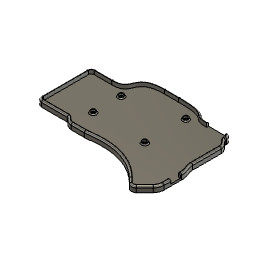
case (Autodesk Fusion 360 design; units mm, degrees)
Autodesk Fusion 360 part; units mm, degrees
note: some values were not read from the file. Chosen so that the rebuilt part matches the saved one: which bodies a step acts on; which pieces of a blend or face edit are solid. Set by a fixed rule: which sketch regions a step uses; the direction of a hole.
sketch "holes" plane through (0, 0, 0) normal (0, 1, 0) x (1, 0, 0)
  line L0 (126.0404, -106.5892) -> (126.0404, -96.5892)
  line L1 (157.8502, -159.4086) -> (150.6767, -159.4086)
  line L2 (126.0404, -96.5892) -> (146.0404, -96.5892)
  line L3 (150.6767, -159.4086) -> (150.6767, -169.4086)
  line L4 (146.0404, -106.5892) -> (126.0404, -106.5892)
  line L5 (150.6767, -169.4086) -> (157.8502, -169.4086)
  line L6 (146.0404, -96.5892) -> (146.0404, -106.5892)
  circle A0 centre (145.3008, -163.4257) radius 0.6
  circle A1 centre (145.3008, -165.1757) radius 0.6
  circle A2 centre (54.3208, -145.8157) radius 2.5
  circle A3 centre (108.3208, -146.3157) radius 2.5
  circle A4 centre (54.3208, -116.8157) radius 2.5
  line L7 (38.8208, -162.5657) -> (47.1808, -162.5657)
  spline S0 degree 3 poles (47.1808, -162.5657) (51.7408, -162.5657) (51.7408, -167.5657) (56.3208, -167.5657) knots 1 1 1 1 2 2 2 2
  line L8 (56.3208, -167.5657) -> (69.8508, -167.5657)
  spline S1 degree 3 poles (69.8508, -167.5657) (75.9008, -167.5657) (75.8208, -166.3157) (88.3208, -166.3157) (106.4584, -166.3157) (123.8522, -173.5257) (136.6708, -186.3576) knots 3 3 3 3 4 4 4 5 5 5 5
  line L9 (136.6708, -186.3576) -> (141.4208, -191.1076)
  spline S2 degree 3 poles (141.4208, -191.1076) (142.2162, -191.8832) (143.4896, -191.8677) (144.266, -191.073) knots 6 6 6 6 7 7 7 7
  line L10 (144.266, -191.073) -> (153.0169, -182.3192)
  spline S3 degree 3 poles (153.0169, -182.3192) (154.5362, -180.8058) (155.392, -178.7508) (155.3961, -176.6064) knots 8 8 8 8 9 9 9 9
  line L11 (155.3961, -176.6064) -> (155.3961, -158.2827)
  spline S4 degree 3 poles (155.3961, -158.2827) (155.3961, -150.8157) (152.3208, -150.8157) (152.3208, -143.8257) knots 10 10 10 10 11 11 11 11
  line L12 (152.3208, -143.8257) -> (152.3208, -114.1112)
  spline S5 degree 3 poles (152.3208, -114.1112) (152.3208, -110.3657) (146.8208, -108.1957) (146.8208, -104.4757) knots 12 12 12 12 13 13 13 13
  line L13 (146.8208, -104.4757) -> (146.8208, -103.0657)
  spline S6 degree 3 poles (146.8208, -103.0657) (146.8208, -101.9611) (145.9254, -101.0657) (144.8208, -101.0657) knots 14 14 14 14 15 15 15 15
  line L14 (144.8208, -101.0657) -> (126.8208, -101.0657)
  spline S7 degree 3 poles (126.8208, -101.0657) (106.3208, -101.0657) (123.3208, -93.0657) (89.0708, -93.0657) knots 17 17 17 17 18 18 18 18
  line L15 (89.0708, -93.0657) -> (74.3308, -93.0657)
  spline S8 degree 3 poles (74.3308, -93.0657) (43.8208, -93.0657) (61.8208, -111.8157) (38.8208, -112.0657) knots 19 19 19 19 20 20 20 20
  spline S9 degree 3 poles (38.8208, -112.0657) (37.7162, -112.0657) (36.8208, -112.9611) (36.8208, -114.0657) knots 20 20 20 20 21 21 21 21
  line L16 (36.8208, -114.0657) -> (36.8208, -114.5657)
  spline S10 degree 3 poles (36.8208, -114.5657) (36.8208, -114.8418) (36.5969, -115.0657) (36.0446, -115.0657) (35.8208, -114.8418) (35.8208, -114.5657) knots 23 23 23 23 24 24 25 25 25 25
  line L17 (35.8208, -114.5657) -> (35.8208, -114.0657)
  spline S11 degree 3 poles (35.8208, -114.0657) (35.8208, -112.9611) (34.9253, -112.0657) (33.8208, -112.0657) knots 26 26 26 26 27 27 27 27
  line L18 (33.8208, -112.0657) -> (20.5708, -112.0657)
  spline S12 degree 3 poles (20.5708, -112.0657) (19.4662, -112.0657) (18.5708, -112.9611) (18.5708, -114.0657) knots 29 29 29 29 30 30 30 30
  line L19 (18.5708, -114.0657) -> (18.5708, -160.5657)
  spline S13 degree 3 poles (18.5708, -160.5657) (18.5708, -161.6703) (19.4662, -162.5657) (20.5708, -162.5657) knots 32 32 32 32 33 33 33 33
  line L20 (20.5708, -162.5657) -> (33.8208, -162.5657)
  spline S14 degree 3 poles (33.8208, -162.5657) (34.9253, -162.5657) (35.8208, -161.6703) (35.8208, -160.5657) knots 35 35 35 35 36 36 36 36
  line L21 (35.8208, -160.5657) -> (35.8208, -160.0657)
  spline S15 degree 3 poles (35.8208, -160.0657) (35.8208, -159.7895) (36.0446, -159.5657) (36.5969, -159.5657) (36.8208, -159.7895) (36.8208, -160.0657) knots 38 38 38 38 39 39 40 40 40 40
  line L22 (36.8208, -160.0657) -> (36.8208, -160.5657)
  spline S16 degree 3 poles (36.8208, -160.5657) (36.8208, -161.6703) (37.7162, -162.5657) (38.8208, -162.5657) knots 41 41 41 41 42 42 42 42
  circle A5 centre (108.3208, -103.8157) radius 2.5
  line L23 (150.6767, -159.4086) -> (162.9306, -159.4086)
  line L24 (162.9306, -159.4086) -> (162.9306, -169.4086)
  line L25 (162.9306, -169.4086) -> (150.6767, -169.4086)
  line L26 (150.6767, -169.4086) -> (150.6767, -159.4086)
  dimension "d39" = 10
  constraint horizontal L23
  constraint vertical L24
  constraint horizontal L25
  constraint vertical L26
  measures "d39" distance of L1.end L3.end
extrude "Extrude7" add sketch "holes" along normal blind 4 contours A2 | A3 | A4 | A5 makes body 1 at (110.2359, 2.6667, 144.7087) makes body 2 at (56.8177, 2.6667, 116.9403) makes body 3 at (52.3279, 2.6667, 147.3252) makes body 4 at (106.328, 2.6667, 105.3252)
hole "Hole1" at (108.3208, 0, 103.8157) at (108.3208, 0, 146.3157) at (54.3208, 0, 116.8157) at (54.3208, 0, 145.8157) direction (0, 1, 0) diameter 3.3 end through all bodies 4 1 2 3
sketch "outline" plane through (0, 0, 0) normal (0, 1, 0) x (1, 0, 0)
  line L0 (38.8208, -162.5657) -> (47.1808, -162.5657)
  spline S0 degree 3 poles (47.1808, -162.5657) (51.7408, -162.5657) (51.7408, -167.5657) (56.3208, -167.5657) knots 1 1 1 1 2 2 2 2
  line L1 (56.3208, -167.5657) -> (69.8508, -167.5657)
  spline S1 degree 3 poles (69.8508, -167.5657) (75.9008, -167.5657) (75.8208, -166.3157) (88.3208, -166.3157) (106.4584, -166.3157) (123.8522, -173.5257) (136.6708, -186.3576) knots 3 3 3 3 4 4 4 5 5 5 5
  line L2 (136.6708, -186.3576) -> (141.4208, -191.1076)
  spline S2 degree 3 poles (141.4208, -191.1076) (142.2162, -191.8832) (143.4896, -191.8677) (144.266, -191.073) knots 6 6 6 6 7 7 7 7
  line L3 (144.266, -191.073) -> (153.0169, -182.3192)
  spline S3 degree 3 poles (153.0169, -182.3192) (154.5362, -180.8058) (155.392, -178.7508) (155.3961, -176.6064) knots 8 8 8 8 9 9 9 9
  line L4 (155.3961, -176.6064) -> (155.3961, -158.2827)
  spline S4 degree 3 poles (155.3961, -158.2827) (155.3961, -150.8157) (152.3208, -150.8157) (152.3208, -143.8257) knots 10 10 10 10 11 11 11 11
  line L5 (152.3208, -143.8257) -> (152.3208, -114.1112)
  spline S5 degree 3 poles (152.3208, -114.1112) (152.3208, -110.3657) (146.8208, -108.1957) (146.8208, -104.4757) knots 12 12 12 12 13 13 13 13
  line L6 (146.8208, -104.4757) -> (146.8208, -103.0657)
  spline S6 degree 3 poles (146.8208, -103.0657) (146.8208, -101.9611) (145.9254, -101.0657) (144.8208, -101.0657) knots 14 14 14 14 15 15 15 15
  line L7 (144.8208, -101.0657) -> (126.8208, -101.0657)
  spline S7 degree 3 poles (126.8208, -101.0657) (106.3208, -101.0657) (123.3208, -93.0657) (89.0708, -93.0657) knots 17 17 17 17 18 18 18 18
  line L8 (89.0708, -93.0657) -> (74.3308, -93.0657)
  spline S8 degree 3 poles (74.3308, -93.0657) (43.8208, -93.0657) (61.8208, -111.8157) (38.8208, -112.0657) knots 19 19 19 19 20 20 20 20
  line L9 (33.8208, -112.0657) -> (20.5708, -112.0657)
  spline S9 degree 3 poles (20.5708, -112.0657) (19.4662, -112.0657) (18.5708, -112.9611) (18.5708, -114.0657) knots 29 29 29 29 30 30 30 30
  line L10 (18.5708, -114.0657) -> (18.5708, -160.5657)
  spline S10 degree 3 poles (18.5708, -160.5657) (18.5708, -161.6703) (19.4662, -162.5657) (20.5708, -162.5657) knots 32 32 32 32 33 33 33 33
  line L11 (20.5708, -162.5657) -> (33.8208, -162.5657)
  line L12 (33.2075, -112.0657) -> (38.8208, -112.0657)
  line L13 (33.8208, -162.5657) -> (38.8208, -162.5657)
  line L14 (33.8208, -111.0657) -> (33.2075, -111.0657)
  line L15 (33.2075, -111.0657) -> (20.5708, -111.0657)
  spline S11 degree 3 poles (20.5708, -111.0657) (19.1158, -111.0657) (17.8856, -112.1155) (17.6229, -113.5068) (17.5886, -113.6885) (17.5708, -113.8757) (17.5708, -114.0657) knots 29 29 29 29 29.884494 29.884494 29.884494 30 30 30 30
  line L16 (17.5708, -114.0657) -> (17.5708, -160.5657)
  spline S12 degree 3 poles (17.5708, -160.5657) (17.5708, -162.0207) (18.6206, -163.2509) (20.0119, -163.5135) (20.1936, -163.5478) (20.3808, -163.5657) (20.5708, -163.5657) knots 32 32 32 32 32.884498 32.884498 32.884498 33 33 33 33
  line L17 (20.5708, -163.5657) -> (33.8208, -163.5657)
  line L18 (33.8208, -163.5657) -> (38.8208, -163.5657)
  line L19 (38.8208, -163.5657) -> (47.1808, -163.5657)
  spline S13 degree 3 poles (47.1808, -163.5657) (48.3085, -163.5657) (48.9835, -163.887) (49.642, -164.4001) (50.4384, -165.0206) (51.1393, -165.9942) (52.1346, -166.9007) (52.9597, -167.6523) (54.0467, -168.3358) (55.4931, -168.5158) (55.758, -168.5487) (56.0338, -168.5657) (56.3208, -168.5657) knots 1 1 1 1 1.294508 1.294508 1.294508 1.650658 1.650658 1.650658 1.945925 1.945925 1.945925 2 2 2 2
  line L20 (56.3208, -168.5657) -> (69.8508, -168.5657)
  spline S14 degree 3 poles (69.8508, -168.5657) (72.9079, -168.5657) (74.4974, -168.2473) (76.7213, -167.9425) (78.9987, -167.6304) (82.0303, -167.3157) (88.3208, -167.3157) (106.1934, -167.3157) (123.332, -174.4199) (135.9633, -187.0643) (135.9634, -187.0644) (135.9634, -187.0644) (135.9635, -187.0645) knots 3 3 3 3 3.494066 3.494066 3.494066 4 4 4 5 5 5 5.000005 5.000005 5.000005 5.000005
  line L21 (135.9635, -187.0645) -> (140.7181, -191.8191)
  spline S15 degree 3 poles (140.7181, -191.8191) (140.7196, -191.8206) (140.7211, -191.822) (140.7226, -191.8235) (141.769, -192.8439) (143.39, -192.9515) (144.5545, -192.1347) (144.7039, -192.0299) (144.8456, -191.9102) (144.9769, -191.7763) knots 5.998113 5.998113 5.998113 5.998113 6 6 6 6.88514 6.88514 6.88514 6.998721 6.998721 6.998721 6.998721
  line L22 (144.9769, -191.7763) -> (153.7227, -183.0277)
  spline S16 degree 3 poles (153.7227, -183.0277) (155.4295, -181.3274) (156.3915, -179.0176) (156.3961, -176.6084) knots 8 8 8 8 9 9 9 9
  line L23 (156.3961, -176.6084) -> (156.3961, -158.2827)
  spline S17 degree 3 poles (156.3961, -158.2827) (156.3961, -154.6595) (155.6583, -152.5745) (154.9277, -150.8359) (154.0973, -148.8598) (153.3208, -147.3882) (153.3208, -143.8257) knots 10 10 10 10 10.468015 10.468015 10.468015 11 11 11 11
  line L24 (153.3208, -143.8257) -> (153.3208, -114.1112)
  spline S18 degree 3 poles (153.3208, -114.1112) (153.3208, -112.786) (152.7693, -111.6472) (152.0791, -110.6811) (151.0533, -109.2452) (149.7009, -108.0687) (148.8245, -106.9104) (148.2228, -106.1152) (147.8613, -105.3804) (147.824, -104.6094) (147.8219, -104.5651) (147.8208, -104.5206) (147.8208, -104.4757) knots 12 12 12 12 12.28049 12.28049 12.28049 12.697372 12.697372 12.697372 12.983577 12.983577 12.983577 13 13 13 13
  line L25 (147.8208, -104.4757) -> (147.8208, -103.0657)
  spline S19 degree 3 poles (147.8208, -103.0657) (147.8208, -101.6107) (146.771, -100.3806) (145.3797, -100.1178) (145.198, -100.0835) (145.0108, -100.0657) (144.8208, -100.0657) knots 14 14 14 14 14.884473 14.884473 14.884473 15 15 15 15
  line L26 (144.8208, -100.0657) -> (126.8208, -100.0657)
  spline S20 degree 3 poles (126.8208, -100.0657) (121.7523, -100.0657) (119.0999, -99.5626) (117.4623, -98.8874) (116.1251, -98.336) (115.4039, -97.6675) (114.4113, -96.8381) (113.2699, -95.8843) (111.8048, -94.7851) (109.0878, -93.9402) (105.5061, -92.8264) (99.7356, -92.0657) (89.0708, -92.0657) knots 17 17 17 17 17.250423 17.250423 17.250423 17.454899 17.454899 17.454899 17.690029 17.690029 17.690029 18 18 18 18
  line L27 (89.0708, -92.0657) -> (74.3308, -92.0657)
  spline S21 degree 3 poles (74.3308, -92.0657) (66.5845, -92.0657) (61.7992, -93.2504) (58.614, -95.1518) (55.7658, -96.8519) (54.2787, -99.1282) (53.2052, -101.3108) (52.1265, -103.504) (51.4038, -105.5915) (50.0955, -107.2158) (48.9858, -108.5934) (47.4793, -109.7072) (44.768, -110.399) (43.2154, -110.7951) (41.2693, -111.0387) (38.8153, -111.0657) knots 19 19 19 19 19.250528 19.250528 19.250528 19.474548 19.474548 19.474548 19.699651 19.699651 19.699651 19.890583 19.890583 19.890583 19.99992 19.99992 19.99992 19.99992
  line L28 (33.8208, -111.0657) -> (38.8153, -111.0657)
  line L29 (33.8208, -109.0657) -> (33.2075, -109.0657)
  line L30 (33.2075, -109.0657) -> (20.5708, -109.0657)
  spline S22 degree 3 poles (20.5708, -109.0657) (19.0114, -109.0657) (17.5811, -109.8001) (16.6674, -110.9408) (15.9839, -111.7942) (15.5708, -112.8992) (15.5708, -114.0657) knots 29 29 29 29 29.572066 29.572066 29.572066 30 30 30 30
  line L31 (15.5708, -114.0657) -> (15.5708, -160.5657)
  spline S23 degree 3 poles (15.5708, -160.5657) (15.5708, -162.1251) (16.3052, -163.5553) (17.4459, -164.469) (18.2993, -165.1525) (19.4043, -165.5657) (20.5708, -165.5657) knots 32 32 32 32 32.572067 32.572067 32.572067 33 33 33 33
  line L32 (20.5708, -165.5657) -> (33.8208, -165.5657)
  line L33 (33.8208, -165.5657) -> (38.8208, -165.5657)
  line L34 (38.8208, -165.5657) -> (47.1808, -165.5657)
  spline S24 degree 3 poles (47.1808, -165.5657) (47.688, -165.5657) (47.8737, -165.6431) (48.1151, -165.7774) (48.4028, -165.9376) (48.7834, -166.2787) (49.3278, -166.8702) (49.8963, -167.4878) (50.6207, -168.3704) (51.7764, -169.1716) (52.7523, -169.8483) (54.0732, -170.4038) (55.5517, -170.5327) (55.8041, -170.5547) (56.0607, -170.5657) (56.3208, -170.5657) knots 1 1 1 1 1.214269 1.214269 1.214269 1.469656 1.469656 1.469656 1.736336 1.736336 1.736336 1.961546 1.961546 1.961546 2 2 2 2
  line L35 (56.3208, -170.5657) -> (69.8508, -170.5657)
  spline S25 degree 3 poles (69.8508, -170.5657) (72.4338, -170.5657) (74.1274, -170.3365) (75.7918, -170.0953) (77.5716, -169.8373) (79.3857, -169.5605) (82.9892, -169.4124) (84.4479, -169.3525) (86.1929, -169.3157) (88.3208, -169.3157) (105.6634, -169.3157) (122.2916, -176.2084) (134.5484, -188.4778) (134.5486, -188.478) (134.5487, -188.4781) (134.5489, -188.4783) knots 3 3 3 3 3.399652 3.399652 3.399652 3.827005 3.827005 3.827005 4 4 4 5 5 5 5.000014 5.000014 5.000014 5.000014
  line L36 (134.5489, -188.4783) -> (139.3128, -193.2422)
  spline S26 degree 3 poles (139.3128, -193.2422) (139.3173, -193.2466) (139.3218, -193.251) (139.3263, -193.2554) (140.4462, -194.3475) (141.9878, -194.8213) (143.4428, -194.6413) (144.522, -194.5078) (145.5836, -194.0104) (146.3972, -193.1844) knots 5.994339 5.994339 5.994339 5.994339 6 6 6 6.572671 6.572671 6.572671 6.997422 6.997422 6.997422 6.997422
  line L37 (146.3972, -193.1844) -> (155.1342, -184.4446)
  spline S27 degree 3 poles (155.1342, -184.4446) (157.2163, -182.3705) (158.3904, -179.5511) (158.3961, -176.6122) (158.3961, -176.6112) (158.3961, -176.6103) (158.3961, -176.6093) knots 8 8 8 8 9 9 9 9.000449 9.000449 9.000449 9.000449
  line L38 (158.3961, -176.6093) -> (158.3961, -158.2827)
  spline S28 degree 3 poles (158.3961, -158.2827) (158.3961, -155.6877) (158.041, -153.7085) (157.5429, -152.1232) (157.0982, -150.7078) (156.5863, -149.6588) (156.2204, -148.7487) (155.7705, -147.6297) (155.4579, -146.6828) (155.3516, -144.9064) (155.3318, -144.5755) (155.3208, -144.2167) (155.3208, -143.8257) knots 10 10 10 10 10.312998 10.312998 10.312998 10.592431 10.592431 10.592431 10.936 10.936 10.936 11 11 11 11
  line L39 (155.3208, -143.8257) -> (155.3208, -114.1112)
  spline S29 degree 3 poles (155.3208, -114.1112) (155.3208, -112.7863) (154.9176, -111.584) (154.3986, -110.6212) (153.5996, -109.139) (152.5735, -108.1057) (151.7369, -107.2079) (151.0162, -106.4344) (150.4285, -105.7668) (150.1283, -105.2841) (149.8952, -104.9093) (149.8367, -104.6932) (149.8236, -104.5414) (149.8217, -104.5195) (149.8208, -104.4981) (149.8208, -104.4757) knots 12 12 12 12 12.198273 12.198273 12.198273 12.503487 12.503487 12.503487 12.766436 12.766436 12.766436 12.970663 12.970663 12.970663 13 13 13 13
  line L40 (149.8208, -104.4757) -> (149.8208, -103.0657)
  spline S30 degree 3 poles (149.8208, -103.0657) (149.8208, -101.5063) (149.0863, -100.076) (147.9455, -99.1623) (147.0922, -98.4788) (145.9872, -98.0657) (144.8208, -98.0657) knots 14 14 14 14 14.57208 14.57208 14.57208 15 15 15 15
  line L41 (144.8208, -98.0657) -> (126.8208, -98.0657)
  spline S31 degree 3 poles (126.8208, -98.0657) (123.1633, -98.0657) (120.874, -97.7898) (119.4474, -97.4322) (118.2335, -97.1279) (117.6573, -96.8152) (117.083, -96.4177) (116.5586, -96.0548) (116.0068, -95.5402) (115.1619, -94.8685) (114.1175, -94.0382) (112.6491, -93.0759) (110.5741, -92.3291) (107.3364, -91.1638) (102.6433, -90.3827) (94.4906, -90.1407) (92.8334, -90.0916) (91.0324, -90.0657) (89.0708, -90.0657) knots 17 17 17 17 17.185474 17.185474 17.185474 17.343292 17.343292 17.343292 17.487402 17.487402 17.487402 17.665535 17.665535 17.665535 17.943497 17.943497 17.943497 18 18 18 18
  line L42 (89.0708, -90.0657) -> (74.3308, -90.0657)
  spline S32 degree 3 poles (74.3308, -90.0657) (68.0798, -90.0657) (63.5856, -90.8058) (60.1525, -92.177) (57.3372, -93.3014) (55.2592, -94.9029) (53.7959, -96.6538) (52.171, -98.5981) (51.2925, -100.6321) (50.538, -102.3109) (49.8536, -103.8339) (49.2673, -105.0606) (48.5263, -105.9756) (47.8592, -106.7994) (47.0963, -107.4409) (45.7016, -108.001) (44.247, -108.5852) (42.0626, -109.0289) (38.8042, -109.0657) knots 19 19 19 19 19.196948 19.196948 19.196948 19.358457 19.358457 19.358457 19.537797 19.537797 19.537797 19.700508 19.700508 19.700508 19.846986 19.846986 19.846986 19.99975 19.99975 19.99975 19.99975
  line L43 (33.8208, -109.0657) -> (38.8042, -109.0657)
  dimension "d42" = 1
  dimension "d43" = 3
  constraint coincident L9 L12.start
  constraint parallel L9 L12
extrude "Extrude8" add sketch "outline" along normal blind 6 separate body contours L29 L30 S22 L31 S23 L32 L33 L34 S24 L35 S25 L36 S26 L37 S27 L38 S28 L39 S29 L40 S30 L41 S31 L42 S32 L43 makes body 5
extrude "Extrude9" add sketch "outline" along normal blind 2 contours L0 S0 L1 S1 L2 S2 L3 S3 L4 S4 L5 S5 L6 S6 L7 S7 L8 S8 L9 S9 L10 S10 L11 L12 L13 | L14 L15 S11 L16 S12 L17 L18 L19 S13 L20 S14 L21 S15 L22 S16 L23 S17 L24 S18 L25 S19 L26 S20 L27 S21 L28 bodies 4 5 1 2 3
extrude "Extrude11" cut sketch "holes" along normal blind 20 from surface at 2 contours L0 L4 L6 S6 L14 S7 | L0 L2 L6 S6 L14 S7 | L1 L3 L5 L11 L23 L25 L26 | L1 L5 L11 L23 L24 L25 bodies 4
chamfer "Chamfer2" distance 1 angle 45 4 edges at (51.99, 2, 117.7197) (51.99, 2, 146.7197) (105.99, 2, 147.2197) (105.99, 2, 104.7197) on bodies 4
fillet "Fillet3" radius 1.8 22 edges at (29.6875, 6, 109.0657) (17.0366, 6, 110.5297) (15.5708, 6, 137.3157) (17.0348, 6, 164.0999) (33.8758, 6, 165.5657) (49.5283, 6, 167.0908) (63.0858, 6, 170.5657) (88.3212, 6, 169.3157) (136.9309, 6, 190.8603) (114.8058, 6, 94.5933) (81.7008, 6, 90.0657) (51.0391, 6, 101.2025) (142.854, 6, 194.6786) (150.7657, 6, 188.8145) (157.5446, 6, 180.8509) (158.3961, 6, 173.009) (158.3961, 6, 158.8456) (156.6237, 6, 149.7056) (155.3208, 6, 128.9684) (151.7657, 6, 107.2387) (149.8208, 6, 103.7707) (148.7466, 6, 99.9722) on bodies 4
named bodies: "case"
